Autodesk Fusion 360 part; units mm, degrees
note: some values were not read from the file. Set by a fixed rule: which face or edge a step refers to.
(part 2 of 2)
sketch "Sketch8" plane through (0, 0, 2) normal (0, 0, 1) x (-1, 0, 0)
  spline S0 degree 5 poles (-35.6583, 21.5031) (-35.6382, 21.2747) (-35.6175, 20.79) (-35.6416, 19.9829) (-35.7623, 18.7701) (-35.9904, 17.1109) (-36.2225, 15.4073) (-36.396, 13.761) (-36.4737, 12.2657) (-36.4561, 10.9952) (-36.3983, 9.9919) (-36.4181, 9.2569) (-36.6442, 8.7697) (-37.1758, 8.5026) (-38.0253, 8.4401) (-39.1167, 8.5824) (-40.3268, 8.9348) (-41.5159, 9.5012) (-42.5593, 10.2767) (-43.3857, 11.2382) (-43.9766, 12.3468) (-44.3458, 13.5544) (-44.527, 14.8101) (-44.5568, 16.0656) (-44.4604, 17.2817) (-44.2369, 18.4338) (-43.8719, 19.507) (-43.3471, 20.4921) (-42.6515, 21.3812) (-41.7915, 22.1639) (-40.8032, 22.8222) (-39.7456, 23.3319) (-38.69, 23.664) (-37.7104, 23.7866) (-36.8738, 23.6669) (-36.2298, 23.2718) (-35.8912, 22.7156) (-35.7385, 22.1603) (-35.6785, 21.7315) (-35.6583, 21.5031) knots 0 0 0 0 0 0 0.028571 0.057143 0.085714 0.114286 0.142857 0.171429 0.2 0.228571 0.257143 0.285714 0.314286 0.342857 0.371429 0.4 0.428571 0.457143 0.485714 0.514286 0.542857 0.571429 0.6 0.628571 0.657143 0.685714 0.714286 0.742857 0.771429 0.8 0.828571 0.857143 0.885714 0.914286 0.942857 0.971429 1 1 1 1 1 1
  line L0 (-21.9822, -3.4637) -> (-21.9822, -2.3506)
  line L1 (-21.9822, -2.3506) -> (-13.3165, -2.3506)
  line L2 (-13.3165, -2.3506) -> (-13.3165, -3.4637)
  line L3 (-13.3165, -3.4637) -> (-21.9822, -3.4637)
  line L4 (5.4476, 10.3439) -> (4.4914, 10.5669)
  line L5 (4.4914, 10.5669) -> (6.0438, 17.223)
  line L6 (6.0438, 17.223) -> (7, 17)
  line L7 (7, 17) -> (5.4476, 10.3439)
  line L8 (12.5139, 0.0359) -> (12.2056, 0.9092)
  line L9 (12.2056, 0.9092) -> (17.8717, 2.909)
  line L10 (17.8717, 2.909) -> (18.1799, 2.0357)
  line L11 (18.1799, 2.0357) -> (12.5139, 0.0359)
  line L12 (21.1796, -1.2973) -> (13.1805, -2.4638)
  line L13 (13.1805, -2.4638) -> (13.0186, -1.3541)
  line L14 (13.0186, -1.3541) -> (21.0177, -0.1875)
  line L15 (21.0177, -0.1875) -> (21.1796, -1.2973)
  line L16 (0.3601, 11) -> (-0.3601, 11)
  line L17 (-0.3601, 11) -> (-0.3601, 17)
  line L18 (-0.3601, 17) -> (0.3601, 17)
  line L19 (0.3601, 17) -> (0.3601, 11)
  line L20 (-20.3157, -9.1297) -> (-20.7229, -8.29)
  line L21 (-20.7229, -8.29) -> (-15.2235, -5.6236)
  line L22 (-15.2235, -5.6236) -> (-14.8164, -6.4634)
  line L23 (-14.8164, -6.4634) -> (-20.3157, -9.1297)
  spline S1 degree 5 poles (34.8518, 21.945) (34.9371, 22.1288) (35.1387, 22.4685) (35.5341, 22.8896) (36.2321, 23.2594) (37.3009, 23.3842) (38.455, 23.1732) (39.5876, 22.6474) (40.6282, 21.8488) (41.5406, 20.8348) (42.3078, 19.6714) (42.9223, 18.4255) (43.3734, 17.159) (43.6362, 15.9211) (43.6617, 14.7424) (43.3986, 13.643) (42.8126, 12.6378) (41.9049, 11.7438) (40.7346, 10.9863) (39.431, 10.404) (38.1528, 10.0401) (37.0546, 9.9359) (36.251, 10.1229) (35.7794, 10.6158) (35.5694, 11.4052) (35.4956, 12.4614) (35.4246, 13.7375) (35.2626, 15.1718) (35.0077, 16.6911) (34.7263, 18.2148) (34.5218, 19.6611) (34.5096, 20.6933) (34.6267, 21.3657) (34.7664, 21.7612) (34.8518, 21.945) knots -1 -1 -1 -1 -1 -1 -0.966667 -0.933333 -0.9 -0.866667 -0.833333 -0.8 -0.766667 -0.733333 -0.7 -0.666667 -0.633333 -0.6 -0.566667 -0.533333 -0.5 -0.466667 -0.433333 -0.4 -0.366667 -0.333333 -0.3 -0.266667 -0.233333 -0.2 -0.166667 -0.133333 -0.1 -0.066667 -0.033333 0 0 0 0 0 0
  spline S2 degree 3 poles (11.2154, -53.2851) (10.1891, -52.8736) (9.3812, -52.0952) (8.9287, -51.2214) (8.3511, -50.1058) (8.2693, -48.9088) (8.4279, -47.8741) (8.5923, -46.8016) (9.0621, -45.8338) (9.8205, -45.1515) (10.7113, -44.3499) (11.874, -43.9685) (13.1906, -43.8196) (14.6835, -43.6506) (16.4477, -43.8051) (18.0295, -44.4868) (19.0286, -44.9174) (19.9643, -45.5592) (20.5382, -46.5227) (20.9518, -47.2172) (21.1279, -48.1015) (20.9526, -48.9383) (20.6952, -50.1674) (19.8008, -51.2026) (18.6612, -51.993) (16.54, -53.4644) (13.4667, -54.1879) (11.2154, -53.2851) knots 0 0 0 0 0.081939 0.081939 0.081939 0.186549 0.186549 0.186549 0.294968 0.294968 0.294968 0.422324 0.422324 0.422324 0.566743 0.566743 0.566743 0.657963 0.657963 0.657963 0.723707 0.723707 0.723707 0.820264 0.820264 0.820264 1 1 1 1
  line L24 (-23.1494, 2.2004) -> (-22.8155, 3.2022)
  line L25 (-22.8155, 3.2022) -> (-12.8166, -0.1308)
  line L26 (-12.8166, -0.1308) -> (-13.1505, -1.1325)
  line L27 (-13.1505, -1.1325) -> (-23.1494, 2.2004)
  line L28 (-2.9359, 4.5075) -> (5, 4.5075)
  line L29 (5, 4.5075) -> (1.0321, -2.1031)
  line L30 (1.0321, -2.1031) -> (-2.9359, 4.5075)
  line L31 (-30.4409, 24.361) -> (-36.9696, -52.963)
  line L32 (-36.9696, -52.963) -> (-39.5943, -52.7414)
  line L33 (-39.5943, -52.7414) -> (-32.6577, 29.4135)
  line L34 (-32.6577, 29.4135) -> (-22.0361, 21.1764)
  line L35 (-22.0361, 21.1764) -> (23.0515, 21.1764)
  line L36 (23.0515, 21.1764) -> (31.7222, 29.4135)
  line L37 (31.7222, 29.4135) -> (41.26, -51.4408)
  line L38 (41.26, -51.4408) -> (38.6441, -51.7494)
  line L39 (38.6441, -51.7494) -> (29.7226, 23.8806)
  line L40 (29.7226, 23.8806) -> (24.1033, 18.5423)
  line L41 (24.1033, 18.5423) -> (-22.9378, 18.5423)
  line L42 (-22.9378, 18.5423) -> (-30.4409, 24.361)
  line L43 (20.277, -7.5382) -> (13.4445, -6.0384)
  line L44 (13.4445, -6.0384) -> (13.6804, -4.9636)
  line L45 (13.6804, -4.9636) -> (20.513, -6.4634)
  line L46 (20.513, -6.4634) -> (20.277, -7.5382)
  line L47 (-4.9671, 10.4674) -> (-6.0248, 10.3131)
  line L48 (-6.0248, 10.3131) -> (-7, 17)
  line L49 (-7, 17) -> (-5.9422, 17.1543)
  line L50 (-5.9422, 17.1543) -> (-4.9671, 10.4674)
  spline S3 degree 3 poles (-23.618, -54.0288) (-24.6321, -53.5076) (-25.4512, -52.8096) (-25.9214, -51.918) (-26.3785, -51.051) (-26.4708, -50.0971) (-26.3342, -49.1764) (-26.1607, -48.0066) (-25.6061, -46.7825) (-24.5794, -45.7973) (-23.479, -44.7413) (-21.8273, -44.0438) (-20.0498, -44.0457) (-18.4067, -44.0474) (-16.6687, -44.6567) (-15.3552, -45.8026) (-14.1282, -46.873) (-13.2824, -48.3807) (-13.1232, -49.9494) (-13.0056, -51.1089) (-13.2923, -52.3202) (-14.0125, -53.2483) (-14.7306, -54.1736) (-15.8211, -54.7492) (-16.9546, -55.0029) (-18.6257, -55.377) (-20.4277, -55.1525) (-21.9392, -54.6967) (-22.5477, -54.5132) (-23.1108, -54.2894) (-23.618, -54.0288) knots 0 0 0 0 0.0968 0.0968 0.0968 0.190927 0.190927 0.190927 0.310527 0.310527 0.310527 0.438722 0.438722 0.438722 0.557218 0.557218 0.557218 0.667914 0.667914 0.667914 0.749733 0.749733 0.749733 0.831315 0.831315 0.831315 0.951586 0.951586 0.951586 1 1 1 1
  spline S4 degree 3 poles (36.2756, 24.4818) (35.9129, 27.8109) (34.9078, 30.65) (33.2588, 33.1044) (31.2853, 36.0416) (28.3419, 38.4643) (24.3484, 40.3397) (20.511, 42.1419) (15.7001, 43.4086) (10.3612, 44.0838) (3.6489, 44.9326) (-3.859, 44.851) (-10.7481, 43.9282) (-16.8751, 43.1075) (-22.4736, 41.6185) (-26.7469, 39.6189) (-30.401, 37.909) (-33.0754, 35.8449) (-34.7789, 33.5483) (-36.5566, 31.1514) (-37.3708, 28.4905) (-37.2774, 25.28) knots -1 -1 -1 -1 -0.879885 -0.879885 -0.879885 -0.73614 -0.73614 -0.73614 -0.598011 -0.598011 -0.598011 -0.42435 -0.42435 -0.42435 -0.269899 -0.269899 -0.269899 -0.137831 -0.137831 -0.137831 0 0 0 0
  line L51 (-37.2774, 25.28) -> (-39.4847, 25.2158)
  spline S5 degree 5 poles (-39.4847, 25.2158) (-39.5154, 26.2725) (-39.4254, 28.3267) (-38.836, 31.2302) (-37.135, 34.7436) (-33.4717, 38.5201) (-28.3084, 41.6536) (-21.7746, 44.1099) (-14.1533, 45.8544) (-5.8392, 46.8513) (2.7148, 47.0639) (11.041, 46.4564) (18.7049, 44.9989) (25.3459, 42.6719) (30.7407, 39.4783) (34.7923, 35.4391) (36.9395, 31.5511) (37.9405, 28.275) (38.3388, 25.9321) (38.4708, 24.7209) knots 0 0 0 0 0 0 0.066667 0.133333 0.2 0.266667 0.333333 0.4 0.466667 0.533333 0.6 0.666667 0.733333 0.8 0.866667 0.933333 1 1 1 1 1 1
  line L52 (38.4708, 24.7209) -> (36.2756, 24.4818)
  line L53 (48, 56.624) -> (48, 64.624)
  line L54 (48, 64.624) -> (-48, 64.624)
  line L55 (-48, 64.624) -> (-48, 56.624)
  line L56 (-48, 56.624) -> (-50.828, 56.624)
  line L57 (-50.828, 56.624) -> (-50.828, -64.624)
  line L58 (-50.828, -64.624) -> (50.828, -64.624)
  line L59 (50.828, -64.624) -> (50.828, 56.624)
  line L60 (50.828, 56.624) -> (48, 56.624)
  line L61 (-18.3094, 10.9644) -> (-12.3137, 7.7359)
  arc A0 (-18.3094, 10.9644) -> (-12.3137, 7.7359) centre (-15.3116, 9.3501) ccw
  line L62 (12.7451, 8.0434) -> (18.2795, 11.4256)
  arc A1 (12.7451, 8.0434) -> (18.2795, 11.4256) centre (15.5123, 9.7345) ccw
extrude "Extrude8" cut sketch "Sketch8" against normal blind 10 contours L61 A0 | L62 A1
sketch "Sketch9" plane through (0, 0, 2) normal (0, 0, 1) x (-1, 0, 0)
  line L0 (12.7451, 8.0434) -> (18.2795, 11.4256)
  arc A0 (12.7451, 8.0434) -> (18.2795, 11.4256) centre (15.5123, 9.7345) ccw
  line L1 (-18.3094, 10.9644) -> (-12.3137, 7.7359)
  arc A1 (-18.3094, 10.9644) -> (-12.3137, 7.7359) centre (-15.3116, 9.3501) ccw
  spline S0 degree 5 poles (-35.6583, 21.5031) (-35.6382, 21.2747) (-35.6175, 20.79) (-35.6416, 19.9829) (-35.7623, 18.7701) (-35.9904, 17.1109) (-36.2225, 15.4073) (-36.396, 13.761) (-36.4737, 12.2657) (-36.4561, 10.9952) (-36.3983, 9.9919) (-36.4181, 9.2569) (-36.6442, 8.7697) (-37.1758, 8.5026) (-38.0253, 8.4401) (-39.1167, 8.5824) (-40.3268, 8.9348) (-41.5159, 9.5012) (-42.5593, 10.2767) (-43.3857, 11.2382) (-43.9766, 12.3468) (-44.3458, 13.5544) (-44.527, 14.8101) (-44.5568, 16.0656) (-44.4604, 17.2817) (-44.2369, 18.4338) (-43.8719, 19.507) (-43.3471, 20.4921) (-42.6515, 21.3812) (-41.7915, 22.1639) (-40.8032, 22.8222) (-39.7456, 23.3319) (-38.69, 23.664) (-37.7104, 23.7866) (-36.8738, 23.6669) (-36.2298, 23.2718) (-35.8912, 22.7156) (-35.7385, 22.1603) (-35.6785, 21.7315) (-35.6583, 21.5031) knots 0 0 0 0 0 0 0.028571 0.057143 0.085714 0.114286 0.142857 0.171429 0.2 0.228571 0.257143 0.285714 0.314286 0.342857 0.371429 0.4 0.428571 0.457143 0.485714 0.514286 0.542857 0.571429 0.6 0.628571 0.657143 0.685714 0.714286 0.742857 0.771429 0.8 0.828571 0.857143 0.885714 0.914286 0.942857 0.971429 1 1 1 1 1 1
  line L2 (-21.9822, -3.4637) -> (-21.9822, -2.3506)
  line L3 (-21.9822, -2.3506) -> (-13.3165, -2.3506)
  line L4 (-13.3165, -2.3506) -> (-13.3165, -3.4637)
  line L5 (-13.3165, -3.4637) -> (-21.9822, -3.4637)
  line L6 (5.4476, 10.3439) -> (4.4914, 10.5669)
  line L7 (4.4914, 10.5669) -> (6.0438, 17.223)
  line L8 (6.0438, 17.223) -> (7, 17)
  line L9 (7, 17) -> (5.4476, 10.3439)
  line L10 (12.5139, 0.0359) -> (12.2056, 0.9092)
  line L11 (12.2056, 0.9092) -> (17.8717, 2.909)
  line L12 (17.8717, 2.909) -> (18.1799, 2.0357)
  line L13 (18.1799, 2.0357) -> (12.5139, 0.0359)
  line L14 (21.1796, -1.2973) -> (13.1805, -2.4638)
  line L15 (13.1805, -2.4638) -> (13.0186, -1.3541)
  line L16 (13.0186, -1.3541) -> (21.0177, -0.1875)
  line L17 (21.0177, -0.1875) -> (21.1796, -1.2973)
  line L18 (0.3601, 11) -> (-0.3601, 11)
  line L19 (-0.3601, 11) -> (-0.3601, 17)
  line L20 (-0.3601, 17) -> (0.3601, 17)
  line L21 (0.3601, 17) -> (0.3601, 11)
  line L22 (-20.3157, -9.1297) -> (-20.7229, -8.29)
  line L23 (-20.7229, -8.29) -> (-15.2235, -5.6236)
  line L24 (-15.2235, -5.6236) -> (-14.8164, -6.4634)
  line L25 (-14.8164, -6.4634) -> (-20.3157, -9.1297)
  spline S1 degree 5 poles (34.8518, 21.945) (34.9371, 22.1288) (35.1387, 22.4685) (35.5341, 22.8896) (36.2321, 23.2594) (37.3009, 23.3842) (38.455, 23.1732) (39.5876, 22.6474) (40.6282, 21.8488) (41.5406, 20.8348) (42.3078, 19.6714) (42.9223, 18.4255) (43.3734, 17.159) (43.6362, 15.9211) (43.6617, 14.7424) (43.3986, 13.643) (42.8126, 12.6378) (41.9049, 11.7438) (40.7346, 10.9863) (39.431, 10.404) (38.1528, 10.0401) (37.0546, 9.9359) (36.251, 10.1229) (35.7794, 10.6158) (35.5694, 11.4052) (35.4956, 12.4614) (35.4246, 13.7375) (35.2626, 15.1718) (35.0077, 16.6911) (34.7263, 18.2148) (34.5218, 19.6611) (34.5096, 20.6933) (34.6267, 21.3657) (34.7664, 21.7612) (34.8518, 21.945) knots -1 -1 -1 -1 -1 -1 -0.966667 -0.933333 -0.9 -0.866667 -0.833333 -0.8 -0.766667 -0.733333 -0.7 -0.666667 -0.633333 -0.6 -0.566667 -0.533333 -0.5 -0.466667 -0.433333 -0.4 -0.366667 -0.333333 -0.3 -0.266667 -0.233333 -0.2 -0.166667 -0.133333 -0.1 -0.066667 -0.033333 0 0 0 0 0 0
  spline S2 degree 3 poles (11.2154, -53.2851) (10.1891, -52.8736) (9.3812, -52.0952) (8.9287, -51.2214) (8.3511, -50.1058) (8.2693, -48.9088) (8.4279, -47.8741) (8.5923, -46.8016) (9.0621, -45.8338) (9.8205, -45.1515) (10.7113, -44.3499) (11.874, -43.9685) (13.1906, -43.8196) (14.6835, -43.6506) (16.4477, -43.8051) (18.0295, -44.4868) (19.0286, -44.9174) (19.9643, -45.5592) (20.5382, -46.5227) (20.9518, -47.2172) (21.1279, -48.1015) (20.9526, -48.9383) (20.6952, -50.1674) (19.8008, -51.2026) (18.6612, -51.993) (16.54, -53.4644) (13.4667, -54.1879) (11.2154, -53.2851) knots 0 0 0 0 0.081939 0.081939 0.081939 0.186549 0.186549 0.186549 0.294968 0.294968 0.294968 0.422324 0.422324 0.422324 0.566743 0.566743 0.566743 0.657963 0.657963 0.657963 0.723707 0.723707 0.723707 0.820264 0.820264 0.820264 1 1 1 1
  line L26 (-23.1494, 2.2004) -> (-22.8155, 3.2022)
  line L27 (-22.8155, 3.2022) -> (-12.8166, -0.1308)
  line L28 (-12.8166, -0.1308) -> (-13.1505, -1.1325)
  line L29 (-13.1505, -1.1325) -> (-23.1494, 2.2004)
  line L30 (-2.9359, 4.5075) -> (5, 4.5075)
  line L31 (5, 4.5075) -> (1.0321, -2.1031)
  line L32 (1.0321, -2.1031) -> (-2.9359, 4.5075)
  line L33 (-30.4409, 24.361) -> (-36.9696, -52.963)
  line L34 (-36.9696, -52.963) -> (-39.5943, -52.7414)
  line L35 (-39.5943, -52.7414) -> (-32.6577, 29.4135)
  line L36 (-32.6577, 29.4135) -> (-22.0361, 21.1764)
  line L37 (-22.0361, 21.1764) -> (23.0515, 21.1764)
  line L38 (23.0515, 21.1764) -> (31.7222, 29.4135)
  line L39 (31.7222, 29.4135) -> (41.26, -51.4408)
  line L40 (41.26, -51.4408) -> (38.6441, -51.7494)
  line L41 (38.6441, -51.7494) -> (29.7226, 23.8806)
  line L42 (29.7226, 23.8806) -> (24.1033, 18.5423)
  line L43 (24.1033, 18.5423) -> (-22.9378, 18.5423)
  line L44 (-22.9378, 18.5423) -> (-30.4409, 24.361)
  line L45 (20.277, -7.5382) -> (13.4445, -6.0384)
  line L46 (13.4445, -6.0384) -> (13.6804, -4.9636)
  line L47 (13.6804, -4.9636) -> (20.513, -6.4634)
  line L48 (20.513, -6.4634) -> (20.277, -7.5382)
  line L49 (-4.9671, 10.4674) -> (-6.0248, 10.3131)
  line L50 (-6.0248, 10.3131) -> (-7, 17)
  line L51 (-7, 17) -> (-5.9422, 17.1543)
  line L52 (-5.9422, 17.1543) -> (-4.9671, 10.4674)
  spline S3 degree 3 poles (-23.618, -54.0288) (-24.6321, -53.5076) (-25.4512, -52.8096) (-25.9214, -51.918) (-26.3785, -51.051) (-26.4708, -50.0971) (-26.3342, -49.1764) (-26.1607, -48.0066) (-25.6061, -46.7825) (-24.5794, -45.7973) (-23.479, -44.7413) (-21.8273, -44.0438) (-20.0498, -44.0457) (-18.4067, -44.0474) (-16.6687, -44.6567) (-15.3552, -45.8026) (-14.1282, -46.873) (-13.2824, -48.3807) (-13.1232, -49.9494) (-13.0056, -51.1089) (-13.2923, -52.3202) (-14.0125, -53.2483) (-14.7306, -54.1736) (-15.8211, -54.7492) (-16.9546, -55.0029) (-18.6257, -55.377) (-20.4277, -55.1525) (-21.9392, -54.6967) (-22.5477, -54.5132) (-23.1108, -54.2894) (-23.618, -54.0288) knots 0 0 0 0 0.0968 0.0968 0.0968 0.190927 0.190927 0.190927 0.310527 0.310527 0.310527 0.438722 0.438722 0.438722 0.557218 0.557218 0.557218 0.667914 0.667914 0.667914 0.749733 0.749733 0.749733 0.831315 0.831315 0.831315 0.951586 0.951586 0.951586 1 1 1 1
  spline S4 degree 3 poles (36.2756, 24.4818) (35.9129, 27.8109) (34.9078, 30.65) (33.2588, 33.1044) (31.2853, 36.0416) (28.3419, 38.4643) (24.3484, 40.3397) (20.511, 42.1419) (15.7001, 43.4086) (10.3612, 44.0838) (3.6489, 44.9326) (-3.859, 44.851) (-10.7481, 43.9282) (-16.8751, 43.1075) (-22.4736, 41.6185) (-26.7469, 39.6189) (-30.401, 37.909) (-33.0754, 35.8449) (-34.7789, 33.5483) (-36.5566, 31.1514) (-37.3708, 28.4905) (-37.2774, 25.28) knots -1 -1 -1 -1 -0.879885 -0.879885 -0.879885 -0.73614 -0.73614 -0.73614 -0.598011 -0.598011 -0.598011 -0.42435 -0.42435 -0.42435 -0.269899 -0.269899 -0.269899 -0.137831 -0.137831 -0.137831 0 0 0 0
  line L53 (-37.2774, 25.28) -> (-39.4847, 25.2158)
  spline S5 degree 5 poles (-39.4847, 25.2158) (-39.5154, 26.2725) (-39.4254, 28.3267) (-38.836, 31.2302) (-37.135, 34.7436) (-33.4717, 38.5201) (-28.3084, 41.6536) (-21.7746, 44.1099) (-14.1533, 45.8544) (-5.8392, 46.8513) (2.7148, 47.0639) (11.041, 46.4564) (18.7049, 44.9989) (25.3459, 42.6719) (30.7407, 39.4783) (34.7923, 35.4391) (36.9395, 31.5511) (37.9405, 28.275) (38.3388, 25.9321) (38.4708, 24.7209) knots 0 0 0 0 0 0 0.066667 0.133333 0.2 0.266667 0.333333 0.4 0.466667 0.533333 0.6 0.666667 0.733333 0.8 0.866667 0.933333 1 1 1 1 1 1
  line L54 (38.4708, 24.7209) -> (36.2756, 24.4818)
  line L55 (48, 56.624) -> (48, 64.624)
  line L56 (48, 64.624) -> (-48, 64.624)
  line L57 (-48, 64.624) -> (-48, 56.624)
  line L58 (-48, 56.624) -> (-50.828, 56.624)
  line L59 (-50.828, 56.624) -> (-50.828, -64.624)
  line L60 (-50.828, -64.624) -> (50.828, -64.624)
  line L61 (50.828, -64.624) -> (50.828, 56.624)
  line L62 (50.828, 56.624) -> (48, 56.624)
  line L63 (21.7186, -58.5) -> (-21.7186, -58.5)
  line L64 (-21.7186, -58.5) -> (-21.7186, -61.5)
  line L65 (-21.7186, -61.5) -> (21.7186, -61.5)
  line L66 (21.7186, -61.5) -> (21.7186, -58.5)
  line L67 (21.7186, -58.5) -> (-21.7186, -61.5) construction
  line L68 (-21.7186, -58.5) -> (21.7186, -61.5) construction
  point P0 (0, -60)
  dimension "d48" = 3
  constraint horizontal L63
  constraint perpendicular L63 L64
  constraint parallel L63 L65
  constraint parallel L64 L66
  constraint coincident L67 P0
  constraint coincident L68 P0
  measures "d48" distance of L63.end L64.end
extrude "Extrude9" add sketch "Sketch9" along normal blind 5 contours L63 L64 L65 L66
fillet "Fillet2" radius 2 2 edges at (21.7186, 60, 7) (-21.7186, 60, 7)
sketch "Sketch10" plane through (0, 61.5, 0) normal (0, 1, 0) x (-1, 0, 0)
  arc A0 (21.7186, 5) -> (19.7186, 7) centre (19.7186, 5) ccw
  line L0 (19.7186, 7) -> (-19.7186, 7)
  arc A1 (-19.7186, 7) -> (-21.7186, 5) centre (-19.7186, 5) ccw
  line L1 (-21.7186, 5) -> (-21.7186, 2)
  line L2 (-21.7186, 2) -> (21.7186, 2)
  line L3 (21.7186, 2) -> (21.7186, 5)
  line L4 (0, 2) -> (0, 4.5)
  line L5 (0, 4.5) -> (17, 4.5)
  line L6 (18, 3.5) -> (18, 2)
  line L7 (18, 2) -> (0, 2)
  line L8 (0, 2) -> (0, 4.5)
  line L9 (0, 4.5) -> (-17, 4.5)
  line L10 (-18, 3.5) -> (-18, 2)
  line L11 (-18, 2) -> (0, 2)
  line L12 (0, 2) -> (0, 4.5)
  arc A2 (-17, 4.5) -> (-18, 3.5) centre (-17, 3.5) ccw
  arc A3 (18, 3.5) -> (17, 4.5) centre (17, 3.5) ccw
  dimension "d53" = 2.5
  dimension "d54" = 1
  constraint midpoint L2 L4.start
  constraint perpendicular L0 L4
  constraint horizontal L5
  constraint vertical L6
  constraint horizontal L7
  constraint vertical L8
  constraint coincident L2 L6.end
  constraint horizontal L9
  constraint vertical L10
  constraint horizontal L11
  constraint vertical L12
  constraint coincident L2 L10.end
  constraint tangent L9 A2
  constraint tangent L10 A2
  constraint tangent L5 A3
  constraint tangent L6 A3
  constraint equal A2 A3
  measures "d53" distance of L4.start L4.end
  measures "d54" radius of A2
extrude "Extrude10" cut sketch "Sketch10" against normal blind 5 contours L2 L4 L5 L6 L7 L8 L12 A3 | L2 L4 L8 L9 L10 L11 L12 A2
extrude "Extrude11" add 1 faces at (-45.3194, -61.2907, -2) along direction (1, 0, 0) blind 1
extrude "Extrude12" add 1 faces at (45.3194, -59.9573, -2) along direction (-1, 0, 0) blind 1
extrude "Extrude13" cut 1 faces at (-48, -60.5743, 1.3298) along direction (1, 0, 0) blind 1
extrude "Extrude14" cut 1 faces at (-50.5, -61.3181, -2.2592) along direction (1, 0, 0) blind 1
extrude "Extrude15" cut 1 faces at (48, -60.5743, 1.3298) along direction (-1, 0, 0) blind 1
extrude "Extrude16" cut 1 faces at (50.5, -61.3181, -2.2592) along direction (-1, 0, 0) blind 1
sketch "Sketch11" plane through (0, 64.624, 0) normal (0, 1, 0) x (-1, 0, 0)
  line L0 (-50.828, 0) -> (50.828, 0)
  line L1 (50.828, 0) -> (50.828, 2)
  line L2 (50.828, 2) -> (-50.828, 2)
  line L3 (-50.828, 2) -> (-50.828, 0)
  line L4 (-50.828, 2) -> (-30.0898, 2)
  line L5 (-30.0898, 2) -> (-30.0941, 0)
  line L6 (-30.0941, 0) -> (-50.828, 0)
  line L7 (-50.828, 0) -> (-50.828, 2)
  constraint horizontal L4
  constraint coincident L0 L5.end
  constraint coincident L2.end L3.start
extrude "Extrude17" add sketch "Sketch11" along normal blind 2 contours L0 L2 L3 L4 L5 L6 L7
mirror "Mirror3" about plane through (0, 0, 0) normal (1, 0, 0) of "Extrude17"
sketch "Sketch12" plane through (0, 66.624, 0) normal (0, 1, 0) x (-1, 0, 0)
  line L0 (-50.828, 0) -> (-30.0941, 0)
  line L1 (-30.0941, 0) -> (-30.0898, 2)
  line L2 (-30.0898, 2) -> (-50.828, 2)
  line L3 (-50.828, 2) -> (-50.828, 0)
  line L4 (-50.828, 0) -> (-30.092, 0)
  line L5 (-30.092, 0) -> (-30.092, 1)
  line L6 (-30.092, 1) -> (-50.828, 1)
  line L7 (-50.828, 1) -> (-50.828, 0)
  constraint horizontal L4
  constraint vertical L5
  constraint horizontal L6
  constraint vertical L7
  constraint midpoint L1 L5.end
  constraint coincident L0.start L3.end
extrude "Extrude18" cut sketch "Sketch12" against normal blind 2 contours L0 L1 L3 L4 L6 L7
mirror "Mirror4" about plane through (0, 0, 0) normal (1, 0, 0) of "Extrude18"
